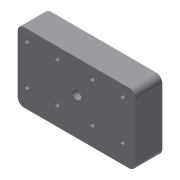
# Autodesk Inventor part: 40_Joystick_PS2_Base
Saved by Autodesk Inventor 2019.4 (Build 234330000, 330)
## iProperties
Created: 2021-10-05
Part Number: 40_Joystick_PS2_Base
Material: Generic
Document SubType Name: Modeling
Designer: diederichbenedict
Density: 1 g/cm^3
Appearance: Default
Author: diederichbenedict
Autodesk Inventor part; units mm, degrees
ref_plane "YZ Plane" through (0, 0, 0) normal (1, 0, 0) x (0, 1, 0)
ref_plane "XZ Plane" through (0, 0, 0) normal (0, 1, 0) x (-1, 0, 0)
ref_plane "Work Plane1" through (0, 0, 0) normal (0, 0, 1) x (1, 0, 0)
ref_plane "Work Plane2" through (0, 0, 2) normal (0, 0, 1) x (1, 0, 0)
sketch "Sketch1" plane through (0, 0, 2) normal (0, 0, 1) x (1, 0, 0)
  circle A0 centre (9.775, 13.7) radius 1.45 construction
  circle A1 centre (-9.775, 13.7) radius 1.45 construction
  circle A2 centre (9.775, -12) radius 1.45 construction
  circle A3 centre (-9.775, -12) radius 1.45 construction
  line L0 (-13.075, -17) -> (13.075, -17) construction
  line L1 (13.075, -17) -> (13.075, 17) construction
  line L2 (13.075, 17) -> (-13.075, 17) construction
  line L3 (-13.075, 17) -> (-13.075, -17) construction
  circle A4 centre (-32.375, 13.7) radius 1.45 construction
  circle A5 centre (-51.925, 13.7) radius 1.45 construction
  circle A6 centre (-32.375, -12) radius 1.45 construction
  circle A7 centre (-51.925, -12) radius 1.45 construction
  line L4 (-55.225, -17) -> (-29.075, -17) construction
  line L5 (-29.075, -17) -> (-29.075, 17) construction
  line L6 (-29.075, 17) -> (-55.225, 17) construction
  line L7 (-55.225, 17) -> (-55.225, -17) construction
  line L8 (18.4, -24.45) -> (-57.6, -24.45) construction
  line L9 (-57.6, -24.45) -> (-57.6, 20.55) construction
  line L10 (-57.6, 20.55) -> (18.4, 20.55) construction
  line L11 (18.4, 20.55) -> (18.4, -24.45) construction
  line L12 (18.4, -24.45) -> (-57.6, 20.55) construction
  line L13 (-57.6, -24.45) -> (18.4, 20.55) construction
  line L14 (18.4, 20.55) -> (-57.6, 20.55)
  line L15 (-57.6, 20.55) -> (-57.6, -24.45)
  line L16 (-57.6, -24.45) -> (18.4, -24.45)
  line L17 (18.4, -24.45) -> (18.4, 20.55)
  circle A8 centre (1.475, 0.05) radius 3.625 projected
  circle A9 centre (-40.675, 0.05) radius 3.625 projected
  point P0 (0, 0)
  point P1 (-19.6, -1.95)
  dimension "d0" = 76
  dimension "d1" = 45
  dimension "d2" = 42.15
  dimension "d3" = 21.075
  dimension "d24" = 2
  constraints: 20 end point, 4 parallel, 2 horizontal, 2 midpoint, 2 perpendicular
  measures "d0" distance of L9.end L10.end
  measures "d1" distance of L8.end L9.end
  measures "d2" distance of A9.centre A8.centre
  measures "d3" horizontal distance of point (-19.6, -1.95) A8.centre
  measures "d24" vertical distance of point (-19.6, -1.95) A9.centre
extrude "Extrusion1" add sketch "Sketch1" along normal blind 2 contours L17 L16 L15 L14 | A8 | A9
sketch "Sketch2" plane through (0, 0, 2) normal (0, 0, -1) x (-1, 0, 0)
  line L0 (48.625, -15.2642) -> (36.125, -15.2642) projected
  line L1 (36.125, -15.2642) -> (36.125, -13.7335) projected
  line L2 (36.125, -13.7335) -> (48.625, -13.7335) projected
  line L3 (48.625, -13.7335) -> (48.625, -15.2642) projected
  line L4 (55.225, -17) -> (29.075, -17) projected
  line L5 (55.225, 17) -> (55.225, -17) projected
  line L6 (29.075, 17) -> (55.225, 17) projected
  line L7 (29.075, -17) -> (29.075, 17) projected
  circle A0 centre (51.925, -12) radius 1.45 projected
  circle A1 centre (32.375, -12) radius 1.45 projected
  circle A2 centre (51.925, 13.7) radius 1.45 projected
  circle A3 centre (32.375, 13.7) radius 1.45 projected
  line L8 (48.025, 8.1) -> (33.325, 8.1) projected
  arc A4 (48.725, 7.4) -> (48.025, 8.1) centre (48.025, 7.4) ccw projected
  line L9 (48.725, 3.55) -> (48.725, 7.4) projected
  line L10 (47.725, 3.55) -> (48.725, 3.55) projected
  line L11 (47.725, -3.45) -> (47.725, 3.55) projected
  line L12 (47.725, -3.45) -> (48.725, -3.45) projected
  line L13 (48.725, -7.3) -> (48.725, -3.45) projected
  arc A5 (48.025, -8) -> (48.725, -7.3) centre (48.025, -7.3) ccw projected
  line L14 (33.325, -8) -> (48.025, -8) projected
  arc A6 (32.625, -7.3) -> (33.325, -8) centre (33.325, -7.3) ccw projected
  line L15 (32.625, 7.4) -> (32.625, -7.3) projected
  arc A7 (33.325, 8.1) -> (32.625, 7.4) centre (33.325, 7.4) ccw projected
  circle A8 centre (51.925, 13.7) radius 3
  circle A9 centre (51.925, -12) radius 3
  circle A10 centre (32.375, -12) radius 3
  circle A11 centre (32.375, 13.7) radius 3
  line L16 (6.475, -15.2642) -> (-6.025, -15.2642) projected
  line L17 (-6.025, -15.2642) -> (-6.025, -13.7335) projected
  line L18 (-6.025, -13.7335) -> (6.475, -13.7335) projected
  line L19 (6.475, -13.7335) -> (6.475, -15.2642) projected
  line L20 (13.075, -17) -> (-13.075, -17) projected
  line L21 (13.075, 17) -> (13.075, -17) projected
  line L22 (-13.075, 17) -> (13.075, 17) projected
  line L23 (-13.075, -17) -> (-13.075, 17) projected
  circle A12 centre (9.775, -12) radius 1.45 projected
  circle A13 centre (-9.775, -12) radius 1.45 projected
  circle A14 centre (9.775, 13.7) radius 1.45 projected
  circle A15 centre (-9.775, 13.7) radius 1.45 projected
  line L24 (5.875, 8.1) -> (-8.825, 8.1) projected
  arc A16 (6.575, 7.4) -> (5.875, 8.1) centre (5.875, 7.4) ccw projected
  line L25 (6.575, 3.55) -> (6.575, 7.4) projected
  line L26 (5.575, 3.55) -> (6.575, 3.55) projected
  line L27 (5.575, -3.45) -> (5.575, 3.55) projected
  line L28 (5.575, -3.45) -> (6.575, -3.45) projected
  line L29 (6.575, -7.3) -> (6.575, -3.45) projected
  arc A17 (5.875, -8) -> (6.575, -7.3) centre (5.875, -7.3) ccw projected
  line L30 (-8.825, -8) -> (5.875, -8) projected
  arc A18 (-9.525, -7.3) -> (-8.825, -8) centre (-8.825, -7.3) ccw projected
  line L31 (-9.525, 7.4) -> (-9.525, -7.3) projected
  arc A19 (-8.825, 8.1) -> (-9.525, 7.4) centre (-8.825, 7.4) ccw projected
  circle A20 centre (9.775, 13.7) radius 3
  circle A21 centre (9.775, -12) radius 3
  circle A22 centre (-9.775, -12) radius 3
  circle A23 centre (-9.775, 13.7) radius 3
  point P0 (0, 0)
  dimension "d6" = 6
  dimension "d7" = 6
  dimension "d8" = 6
  dimension "d9" = 6
  dimension "d10" = 6
  dimension "d11" = 6
  dimension "d12" = 6
  dimension "d13" = 6
  constraints: 8 centre point, 8 coincident
  measures "d6" diameter of A8
  measures "d7" diameter of A9
  measures "d8" diameter of A10
  measures "d9" diameter of A11
  measures "d10" diameter of A20
  measures "d11" diameter of A21
  measures "d12" diameter of A22
  measures "d13" diameter of A23
extrude "Extrusion2" add sketch "Sketch2" along normal blind 2 contours A8 | A9 | A10 | A11 | A20 | A21 | A22 | A23
fillet "Fillet1" radius 4 4 edges at (18.4, 20.55, 3) (18.4, -24.45, 3) (-57.6, -24.45, 3) (-57.6, 20.55, 3)
sketch "Sketch3" plane through (0, 0, 2) normal (0, 0, -1) x (-1, 0, 0)
  circle A0 centre (-9.775, -12) radius 3 projected
  circle A1 centre (9.775, 13.7) radius 3 projected
  circle A2 centre (32.375, -12) radius 3 projected
  circle A3 centre (51.925, 13.7) radius 3 projected
  circle A4 centre (51.925, -12) radius 3 projected
  circle A5 centre (32.375, 13.7) radius 3 projected
  circle A6 centre (9.775, -12) radius 3 projected
  circle A7 centre (-9.775, 13.7) radius 3 projected
  arc A8 (57.6, 16.55) -> (53.6, 20.55) centre (53.6, 16.55) ccw projected
  line L0 (53.6, 20.55) -> (-14.4, 20.55) projected
  arc A9 (-14.4, 20.55) -> (-18.4, 16.55) centre (-14.4, 16.55) ccw projected
  line L1 (-18.4, 16.55) -> (-18.4, -20.45) projected
  arc A10 (-18.4, -20.45) -> (-14.4, -24.45) centre (-14.4, -20.45) ccw projected
  line L2 (-14.4, -24.45) -> (53.6, -24.45) projected
  arc A11 (53.6, -24.45) -> (57.6, -20.45) centre (53.6, -20.45) ccw projected
  line L3 (57.6, -20.45) -> (57.6, 16.55) projected
  point P0 (0, 0)
hole "Hole1" at (-51.925, 13.7, 2) at (-51.925, -12, 2) at (-32.375, -12, 2) at (-32.375, 13.7, 2) at (-9.775, 13.7, 2) at (9.775, 13.7, 2) at (-9.775, -12, 2) at (9.775, -12, 2) direction (0, 0, 1) diameter 2.9 end through all
ref_plane "Work Plane3" through (-11.0937, -12.5187, -13.35) normal (0, 0, 1) x (1, 0, 0)
sketch "Sketch4" plane through (0, 0, 2) normal (0, 0, -1) x (-1, 0, 0)
  circle A0 centre (-9.775, -12) radius 3 projected
  circle A1 centre (9.775, 13.7) radius 3 projected
  circle A2 centre (32.375, -12) radius 3 projected
  circle A3 centre (51.925, 13.7) radius 3 projected
  circle A4 centre (51.925, -12) radius 3 projected
  circle A5 centre (32.375, 13.7) radius 3 projected
  circle A6 centre (9.775, -12) radius 3 projected
  circle A7 centre (-9.775, 13.7) radius 3 projected
  arc A8 (57.6, 16.55) -> (53.6, 20.55) centre (53.6, 16.55) ccw projected
  line L0 (53.6, 20.55) -> (-14.4, 20.55) projected
  arc A9 (-14.4, 20.55) -> (-18.4, 16.55) centre (-14.4, 16.55) ccw projected
  line L1 (-18.4, 16.55) -> (-18.4, -20.45) projected
  arc A10 (-18.4, -20.45) -> (-14.4, -24.45) centre (-14.4, -20.45) ccw projected
  line L2 (-14.4, -24.45) -> (53.6, -24.45) projected
  arc A11 (53.6, -24.45) -> (57.6, -20.45) centre (53.6, -20.45) ccw projected
  line L3 (57.6, -20.45) -> (57.6, 16.55) projected
  arc A12 (55.6, 16.55) -> (53.6, 18.55) centre (53.6, 16.55) ccw
  line L4 (53.6, 18.55) -> (-14.4, 18.55)
  arc A13 (-14.4, 18.55) -> (-16.4, 16.55) centre (-14.4, 16.55) ccw
  line L5 (-16.4, 16.55) -> (-16.4, -20.45)
  arc A14 (-16.4, -20.45) -> (-14.4, -22.45) centre (-14.4, -20.45) ccw
  line L6 (-14.4, -22.45) -> (53.6, -22.45)
  arc A15 (53.6, -22.45) -> (55.6, -20.45) centre (53.6, -20.45) ccw
  line L7 (55.6, -20.45) -> (55.6, 16.55)
  point P0 (0, 0)
  dimension "d25" = 2
  constraints: 8 end point, 8 point on circle, 4 centre point, 7 other
  measures "d25" distance between parallel lines of L3 L7
extrude "Extrusion3" add sketch "Sketch4" along normal up to surface (15.35 mm away) contours L3 A11 L2 A10 L1 A9 L0 A8
sketch "Sketch5" plane through (-53.6, -24.45, 4) normal (0, -1, 0) x (1, 0, 0)
  line L0 (0, -17.35) -> (0, 0) projected
  line L1 (68, 0) -> (68, -17.35) projected
  line L2 (0, 0) -> (68, 0) projected
  circle A0 centre (34, -7) radius 2.5
  line L3 (68, -17.35) -> (0, -17.35) projected
  point P0 (53.6, -4)
  dimension "d28" = 5
  constraints: 1 centre point
  measures "d28" diameter of A0
extrude "Extrusion4" cut sketch "Sketch5" against normal blind 12 contours A0
sketch "Sketch6" plane through (0, 0, -13.35) normal (0, 0, -1) x (-1, 0, 0)
  line L0 (55.6, 16.55) -> (55.6, -20.45) projected
  arc A0 (53.6, -22.45) -> (55.6, -20.45) centre (53.6, -20.45) ccw projected
  line L1 (53.6, -22.45) -> (-14.4, -22.45) projected
  arc A1 (-16.4, -20.45) -> (-14.4, -22.45) centre (-14.4, -20.45) ccw projected
  line L2 (-16.4, -20.45) -> (-16.4, 16.55) projected
  arc A2 (-14.4, 18.55) -> (-16.4, 16.55) centre (-14.4, 16.55) ccw projected
  line L3 (-14.4, 18.55) -> (53.6, 18.55) projected
  arc A3 (55.6, 16.55) -> (53.6, 18.55) centre (53.6, 16.55) ccw projected
  arc A4 (57.6, 16.55) -> (53.6, 20.55) centre (53.6, 16.55) ccw projected
  line L4 (53.6, 20.55) -> (-14.4, 20.55) projected
  arc A5 (-14.4, 20.55) -> (-18.4, 16.55) centre (-14.4, 16.55) ccw projected
  line L5 (-18.4, 16.55) -> (-18.4, -20.45) projected
  arc A6 (-18.4, -20.45) -> (-14.4, -24.45) centre (-14.4, -20.45) ccw projected
  line L6 (-14.4, -24.45) -> (53.6, -24.45) projected
  arc A7 (53.6, -24.45) -> (57.6, -20.45) centre (53.6, -20.45) ccw projected
  line L7 (57.6, -20.45) -> (57.6, 16.55) projected
  line L8 (15.6, 8) -> (23.6, 8)
  line L9 (23.6, 8) -> (23.6, -8)
  line L10 (23.6, -8) -> (15.6, -8)
  line L11 (15.6, -8) -> (15.6, 8)
  line L12 (15.6, 8) -> (23.6, -8) construction
  line L13 (23.6, 8) -> (15.6, -8) construction
  point P0 (0, 0)
  point P1 (19.6, 0)
  dimension "d31" = 8
  dimension "d32" = 16
  constraints: 12 end point, 2 midpoint, 2 parallel, 1 horizontal, 1 perpendicular
  measures "d31" distance of L9.end L10.end
  measures "d32" distance of L8.end L9.end
extrude "Extrusion5" add sketch "Sketch6" against normal up to next contours L8 L9 L10 L11
sketch "Sketch7" plane through (0, 0, 4) normal (0, 0, 1) x (1, 0, 0)
  line L0 (-15.6, 8) -> (-23.6, 8) projected
  line L1 (-15.6, -8) -> (-15.6, 8) projected
  line L2 (-23.6, -8) -> (-15.6, -8) projected
  line L3 (-23.6, 8) -> (-23.6, -8) projected
  circle A0 centre (-19.6, 0) radius 1.5839
  point P0 (0, 0)
  constraints: 1 centre point
hole "Hole2" at (-19.6, 0, 4) direction (0, 0, -1) diameter 2.9 end through all counterbore diameter 6 counterbore depth 3.5
equation "\"d3\" = 0.5 * d2"
body "Solid1"
